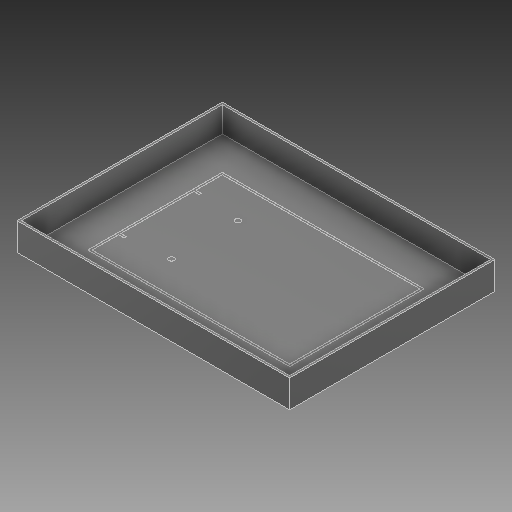
# Autodesk Inventor part: Board_main
Saved by Autodesk Inventor 2023 (Build 270158000, 158)
## iProperties
Created: 2022-01-17
Part Number: Board_main
Material: Типовые
Document SubType Name: Modeling
Designer: Администратор
Density: 1 g/cm^3
Appearance: С гладкой текстурой — черный
Author: Администратор
Autodesk Inventor part; units mm, degrees
ref_plane "YZ Plane" through (0, 0, 0) normal (1, 0, 0) x (0, 1, 0)
ref_plane "XZ Plane" through (0, 0, 0) normal (0, 1, 0) x (-1, 0, 0)
ref_plane "XY Plane" through (0, 0, 0) normal (0, 0, 1) x (1, 0, 0)
sketch "Эскиз1" plane through (0, 0, 0) normal (0, 1, 0) x (-1, 0, 0)
  line L0 (1215, -910) -> (-1215, -910)
  line L1 (-1215, -910) -> (-1215, 910)
  line L2 (-1215, 910) -> (1215, 910)
  line L3 (1215, 910) -> (1215, -910)
  line L4 (0, -910) -> (0, 910) construction
  line L5 (1215, 0) -> (-1215, 0) construction
  line L6 (-1235, -930) -> (1235, -930)
  line L7 (1235, -930) -> (1235, 930)
  line L8 (1235, 930) -> (-1235, 930)
  line L9 (-1235, 930) -> (-1235, -930)
  point P0 (0, 0)
  point P1 (0, 0)
  dimension "d0" = 1820
  dimension "d1" = 2430
  dimension "d2" = 20
  constraints: 20 end point, 5 midpoint, 4 parallel, 2 perpendicular, 1 coincident, 1 horizontal, 3 other
  measures "d0" distance of L2.end L0.start
  measures "d1" distance of L0.start L0.end
  measures "d2" distance between parallel lines of L0 L6
extrude "Выдавливание1" add sketch "Эскиз1" along normal blind 230
extrude "Выдавливание2" add sketch "Эскиз1" against normal blind 20 contours L0 L1 L2 L3 | L9 L8 L7 L6
sketch "Эскиз2" plane through (0, 0, 0) normal (0, 1, 0) x (1, 0, 0)
  line L0 (-1215, -910) -> (-1215, 910) projected
  line L1 (1215, -910) -> (-1215, -910) projected
  line L2 (1215, 910) -> (1215, -910) projected
  line L3 (-1215, 910) -> (1215, 910) projected
  line L4 (915, 610) -> (915, -610)
  line L5 (915, -610) -> (-915, -610)
  line L6 (-915, -610) -> (-915, 610)
  line L7 (-915, 610) -> (915, 610)
  line L8 (-915, 0) -> (915, 0)
  circle A0 centre (-465, 300) radius 25
  circle A1 centre (-465, -300) radius 25
  line L9 (895, 590) -> (895, -590)
  line L10 (895, -590) -> (-895, -590)
  line L11 (-895, -590) -> (-895, 590)
  line L12 (-895, 590) -> (895, 590)
  line L13 (-895, 350) -> (-845, 350)
  line L14 (-845, 350) -> (-845, 330)
  line L15 (-845, 330) -> (-895, 330)
  line L16 (-895, -350) -> (-845, -350)
  line L17 (-845, -350) -> (-845, -330)
  line L18 (-845, -330) -> (-895, -330)
  point P0 (0, 0)
  point P1 (895, 0)
  point P2 (-895, 0)
  point P3 (-895, -330)
  point P4 (-895, -350)
  dimension "d7" = 300
  dimension "d9" = 50
  dimension "d10" = 310
  dimension "d11" = 450
  dimension "d14" = 20
  dimension "d15" = 50
  dimension "d18" = 350
  dimension "d19" = 20
  constraints: 30 end point, 6 symmetric about line, 2 centre point, 2 midpoint, 2 point on line, 1 horizontal, 1 perpendicular, 1 vertical, 11 other
  measures "d7" distance between parallel lines of L3 L7
  measures "d9" diameter of A0
  measures "d10" distance from line of L7 A0.centre
  measures "d11" distance from line of L6 A0.centre
  measures "d14" distance between parallel lines of L7 L12
  measures "d15" distance of L13.start L13.end
  measures "d18" distance between parallel lines of L8 L13
  measures "d19" distance of L13.end L14.end
extrude "Выдавливание3" cut sketch "Эскиз2" against normal blind 1 contours L4 L8 L9 L12 L11 L6 L7 | L4 L5 L6 L8 L11 L10 L9 | L18 L17 L16 L11 | L11 L13 L14 L15 | A0 | A1
